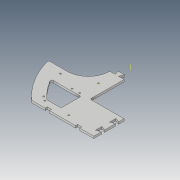
# Autodesk Inventor part: BR_topPlate
Saved by Autodesk Inventor 2018 (Build 220112000, 112)
## iProperties
Created: 2020-01-08
Part Number: BR_topPlate
Material: Generic
Document SubType Name: Modeling
Designer: anirudh
Density: 1 g/cm^3
Appearance: Default
Author: anirudh
Autodesk Inventor part; units mm, degrees
ref_plane "YZ Plane" through (0, 0, 0) normal (1, 0, 0) x (0, 1, 0)
ref_plane "XZ Plane" through (0, 0, 0) normal (0, 1, 0) x (-1, 0, 0)
ref_plane "XY Plane" through (0, 0, 0) normal (0, 0, 1) x (1, 0, 0)
sketch "Sketch1" plane through (0, 0, 0) normal (0, 1, 0) x (-1, 0, 0)
  line L0 (-159.8042, -152.4) -> (-128.1081, -152.4)
  line L1 (-159.8042, -152.4) -> (-128.1081, -152.4)
  line L2 (-128.1081, -147.32) -> (-117.9481, -147.32)
  line L3 (-128.1081, -152.4) -> (-128.1081, -147.32)
  line L4 (-117.9481, -147.32) -> (-117.9481, -152.4)
  line L5 (-128.1081, -147.32) -> (-117.9481, -147.32)
  line L6 (-117.9481, -152.4) -> (-55.88, -152.4)
  line L7 (-117.9481, -147.32) -> (-117.9481, -152.4)
  line L8 (-117.9481, -152.4) -> (-55.88, -152.4)
  line L9 (-55.88, -147.32) -> (-45.72, -147.32)
  line L10 (-55.88, -152.4) -> (-55.88, -147.32)
  line L11 (-45.72, -147.32) -> (-45.72, -152.4)
  line L12 (-55.88, -147.32) -> (-45.72, -147.32)
  line L13 (-45.72, -152.4) -> (20.32, -152.4)
  line L14 (-45.72, -147.32) -> (-45.72, -152.4)
  line L15 (-45.72, -152.4) -> (20.32, -152.4)
  line L16 (20.32, -147.32) -> (30.48, -147.32)
  line L17 (20.32, -152.4) -> (20.32, -147.32)
  line L18 (30.48, -147.32) -> (30.48, -152.4)
  line L19 (20.32, -147.32) -> (30.48, -147.32)
  line L20 (30.48, -147.32) -> (30.48, -152.4)
  line L21 (30.48, -152.4) -> (92.5481, -152.4)
  line L22 (30.48, -152.4) -> (92.5481, -152.4)
  line L23 (92.5481, -147.32) -> (102.7081, -147.32)
  line L24 (92.5481, -152.4) -> (92.5481, -147.32)
  line L25 (102.7081, -147.32) -> (102.7081, -152.4)
  line L26 (92.5481, -147.32) -> (102.7081, -147.32)
  line L27 (102.7081, -147.32) -> (102.7081, -152.4)
  arc A0 (134.4042, -152.4) -> (195.6623, -54.8317) centre (0, 0) ccw
  line L28 (102.7081, -152.4) -> (134.4042, -152.4)
  arc A1 (-221.0623, -54.8317) -> (-159.8042, -152.4) centre (-25.4, 0) ccw
  line L29 (134.4042, 152.4) -> (102.7081, 152.4)
  line L30 (134.4042, 152.4) -> (102.7081, 152.4)
  line L31 (-128.1081, 152.4) -> (-159.8042, 152.4)
  line L32 (-128.1081, 147.32) -> (-128.1081, 152.4)
  line L33 (-159.8042, 152.4) -> (-128.1081, 152.4)
  line L34 (-117.9481, 147.32) -> (-128.1081, 147.32)
  line L35 (-128.1081, 152.4) -> (-128.1081, 147.32)
  line L36 (-128.1081, 147.32) -> (-117.9481, 147.32)
  line L37 (-55.88, 152.4) -> (-117.9481, 152.4)
  line L38 (-117.9481, 147.32) -> (-117.9481, 152.4)
  line L39 (-55.88, 147.32) -> (-55.88, 152.4)
  line L40 (-117.9481, 152.4) -> (-55.88, 152.4)
  line L41 (-45.72, 147.32) -> (-55.88, 147.32)
  line L42 (-55.88, 152.4) -> (-55.88, 147.32)
  line L43 (-55.88, 147.32) -> (-45.72, 147.32)
  line L44 (20.32, 152.4) -> (-45.72, 152.4)
  line L45 (-45.72, 147.32) -> (-45.72, 152.4)
  line L46 (-45.72, 152.4) -> (20.32, 152.4)
  line L47 (30.48, 147.32) -> (20.32, 147.32)
  line L48 (20.32, 152.4) -> (20.32, 147.32)
  line L49 (20.32, 147.32) -> (30.48, 147.32)
  line L50 (30.48, 152.4) -> (30.48, 147.32)
  line L51 (30.48, 147.32) -> (30.48, 152.4)
  line L52 (92.5481, 147.32) -> (92.5481, 152.4)
  line L53 (30.48, 152.4) -> (92.5481, 152.4)
  line L54 (92.5481, 152.4) -> (92.5481, 147.32)
  line L55 (102.7081, 152.4) -> (102.7081, 147.32)
  line L56 (92.5481, 147.32) -> (102.7081, 147.32)
  line L57 (102.7081, 147.32) -> (102.7081, 152.4)
  arc A2 (-177.8, -50.8) -> (-177.8, 50.8) centre (-177.8, 0) ccw
  arc A3 (-177.8, -50.8) -> (-177.8, 50.8) centre (-177.8, 0) ccw
  arc A4 (152.4, 50.8) -> (152.4, -50.8) centre (152.4, 0) ccw
  arc A5 (152.4, 50.8) -> (152.4, -50.8) centre (152.4, 0) ccw
  line L58 (152.4, -50.8) -> (196.7476, -50.8)
  line L59 (152.4, 50.8) -> (196.7476, 50.8)
  line L60 (-177.8, -50.8) -> (-218.005, -50.8)
  line L61 (-177.8, -50.8) -> (-222.1476, -50.8)
  line L62 (-218.005, 50.8) -> (-177.8, 50.8)
  line L63 (-177.8, 50.8) -> (-222.1476, 50.8)
  arc A6 (-159.8042, 152.4) -> (-222.1476, 50.8) centre (-25.4, 0) ccw
  arc A7 (-222.1476, -50.8) -> (-159.8042, -152.4) centre (-25.4, 0) ccw
  arc A8 (134.4042, -152.4) -> (196.7476, -50.8) centre (0, 0) ccw
  arc A9 (196.7476, 50.8) -> (134.4042, 152.4) centre (0, 0) ccw
  line L64 (-12.7, -80.645) -> (-93.345, -80.645)
  line L65 (-93.345, -80.645) -> (67.945, -80.645)
  line L66 (67.945, -80.645) -> (67.945, 80.645)
  line L67 (67.945, 80.645) -> (-93.345, 80.645)
  line L68 (-93.345, 80.645) -> (-93.345, -80.645)
  circle A10 centre (-177.8, -63.5) radius 1.75
  circle A11 centre (-177.8, -63.5) radius 1.75
  circle A12 centre (-177.8, 63.5) radius 1.75
  circle A13 centre (-177.8, 63.5) radius 1.75
  circle A14 centre (-136.1822, -80.3402) radius 1.75
  circle A15 centre (-136.1822, -80.3402) radius 1.75
  circle A16 centre (-118.4022, -80.3402) radius 1.75
  circle A17 centre (-118.4022, -80.3402) radius 1.75
  circle A18 centre (-136.1822, 80.3402) radius 1.75
  circle A19 centre (-136.1822, 80.3402) radius 1.75
  circle A20 centre (-118.4022, 80.3402) radius 1.75
  circle A21 centre (-118.4022, 80.3402) radius 1.75
  circle A22 centre (93.0022, -80.3402) radius 1.75
  circle A23 centre (93.0022, -80.3402) radius 1.75
  circle A24 centre (110.7822, -80.3402) radius 1.75
  circle A25 centre (110.7822, -80.3402) radius 1.75
  circle A26 centre (152.4, -63.5) radius 1.75
  circle A27 centre (152.4, -63.5) radius 1.75
  circle A28 centre (152.4, 63.5) radius 1.75
  circle A29 centre (152.4, 63.5) radius 1.75
  circle A30 centre (93.0022, 80.3402) radius 1.75
  circle A31 centre (93.0022, 80.3402) radius 1.75
  circle A32 centre (110.7822, 80.3402) radius 1.75
  circle A33 centre (110.7822, 80.3402) radius 1.75
  dimension "d4" = 80.645
  dimension "d5" = 161.29
  constraints: 139 end point, 34 centre point, 30 perpendicular, 22 point on circle, 16 coincident, 6 horizontal, 4 collinear, 4 point on line, 2 parallel, 2 tangent
  measures "d4" distance of L64.start L64.end
  measures "d5" distance of L68.start L67.start
extrude "Extrusion1" add sketch "Sketch1" along normal blind 5.08
fillet "Fillet1" radius 3.175 8 edges at (222.1476, 2.54, 50.8) (222.1476, 2.54, -50.8) (93.345, 2.54, 80.645) (93.345, 2.54, -80.645) (-67.945, 2.54, -80.645) (-67.945, 2.54, 80.645) (-196.7476, 2.54, 50.8) (-196.7476, 2.54, -50.8)
sketch "Sketch2" plane through (0, 5.08, 0) normal (0, 1, 0) x (1, 0, 0)
  line L0 (-116.3974, -133.35) -> (-87.2998, -133.35)
  line L1 (-116.3974, -133.35) -> (-87.2998, -133.35)
  line L2 (-84.1248, -130.175) -> (-84.1248, -89.2048)
  line L3 (-84.1248, -130.175) -> (-84.1248, -89.2048)
  line L4 (-87.2998, -86.0298) -> (-150.1213, -86.0298)
  line L5 (-87.2998, -86.0298) -> (-150.1213, -86.0298)
  arc A0 (-152.8507, -90.8267) -> (-118.5137, -132.5418) centre (0, 0) ccw
  arc A1 (-152.8507, -90.8267) -> (-118.5137, -132.5418) centre (0, 0) ccw
  arc A2 (-118.5137, -132.5418) -> (-116.3974, -133.35) centre (-116.3974, -130.175) ccw
  arc A3 (-118.5137, -132.5418) -> (-116.3974, -133.35) centre (-116.3974, -130.175) ccw
  arc A4 (-87.2998, -133.35) -> (-84.1248, -130.175) centre (-87.2998, -130.175) ccw
  arc A5 (-87.2998, -133.35) -> (-84.1248, -130.175) centre (-87.2998, -130.175) ccw
  arc A6 (-84.1248, -89.2048) -> (-87.2998, -86.0298) centre (-87.2998, -89.2048) ccw
  arc A7 (-84.1248, -89.2048) -> (-87.2998, -86.0298) centre (-87.2998, -89.2048) ccw
  arc A8 (-150.1213, -86.0298) -> (-152.8507, -90.8267) centre (-150.1213, -89.2048) ccw
  arc A9 (-150.1213, -86.0298) -> (-152.8507, -90.8267) centre (-150.1213, -89.2048) ccw
  arc A10 (-152.4, -50.8) -> (-152.4, 50.8) centre (-152.4, 0) ccw
  arc A11 (177.8, 50.8) -> (177.8, -50.8) centre (177.8, 0) ccw
  line L6 (141.7974, -133.35) -> (112.6998, -133.35)
  line L7 (141.7974, -133.35) -> (112.6998, -133.35)
  line L8 (109.5248, -130.175) -> (109.5248, -89.2048)
  line L9 (109.5248, -130.175) -> (109.5248, -89.2048)
  line L10 (112.6998, -86.0298) -> (175.5213, -86.0298)
  line L11 (112.6998, -86.0298) -> (175.5213, -86.0298)
  arc A12 (112.6998, -86.0298) -> (109.5248, -89.2048) centre (112.6998, -89.2048) ccw
  arc A13 (112.6998, -86.0298) -> (109.5248, -89.2048) centre (112.6998, -89.2048) ccw
  arc A14 (178.2507, -90.8267) -> (175.5213, -86.0298) centre (175.5213, -89.2048) ccw
  arc A15 (178.2507, -90.8267) -> (175.5213, -86.0298) centre (175.5213, -89.2048) ccw
  arc A16 (109.5248, -130.175) -> (112.6998, -133.35) centre (112.6998, -130.175) ccw
  arc A17 (109.5248, -130.175) -> (112.6998, -133.35) centre (112.6998, -130.175) ccw
  arc A18 (143.9137, -132.5418) -> (178.2507, -90.8267) centre (25.4, 0) ccw
  arc A19 (143.9137, -132.5418) -> (178.2507, -90.8267) centre (25.4, 0) ccw
  arc A20 (141.7974, -133.35) -> (143.9137, -132.5418) centre (141.7974, -130.175) ccw
  arc A21 (141.7974, -133.35) -> (143.9137, -132.5418) centre (141.7974, -130.175) ccw
  arc A22 (-152.4, -50.8) -> (-152.4, 50.8) centre (-152.4, 0) ccw projected
  arc A23 (177.8, 50.8) -> (177.8, -50.8) centre (177.8, 0) ccw projected
  line L12 (-116.3974, 133.35) -> (-87.2998, 133.35)
  line L13 (-116.3974, 133.35) -> (-87.2998, 133.35)
  line L14 (-84.1248, 130.175) -> (-84.1248, 89.2048)
  line L15 (-84.1248, 130.175) -> (-84.1248, 89.2048)
  line L16 (-87.2998, 86.0298) -> (-150.1213, 86.0298)
  line L17 (-87.2998, 86.0298) -> (-150.1213, 86.0298)
  arc A24 (-118.5137, 132.5418) -> (-152.8507, 90.8267) centre (0, 0) ccw
  arc A25 (-118.5137, 132.5418) -> (-152.8507, 90.8267) centre (0, 0) ccw
  arc A26 (-116.3974, 133.35) -> (-118.5137, 132.5418) centre (-116.3974, 130.175) ccw
  arc A27 (-116.3974, 133.35) -> (-118.5137, 132.5418) centre (-116.3974, 130.175) ccw
  arc A28 (-84.1248, 130.175) -> (-87.2998, 133.35) centre (-87.2998, 130.175) ccw
  arc A29 (-84.1248, 130.175) -> (-87.2998, 133.35) centre (-87.2998, 130.175) ccw
  arc A30 (-87.2998, 86.0298) -> (-84.1248, 89.2048) centre (-87.2998, 89.2048) ccw
  arc A31 (-87.2998, 86.0298) -> (-84.1248, 89.2048) centre (-87.2998, 89.2048) ccw
  arc A32 (-152.8507, 90.8267) -> (-150.1213, 86.0298) centre (-150.1213, 89.2048) ccw
  arc A33 (-152.8507, 90.8267) -> (-150.1213, 86.0298) centre (-150.1213, 89.2048) ccw
  line L18 (141.7974, 133.35) -> (112.6998, 133.35)
  line L19 (141.7974, 133.35) -> (112.6998, 133.35)
  line L20 (109.5248, 130.175) -> (109.5248, 89.2048)
  line L21 (109.5248, 130.175) -> (109.5248, 89.2048)
  line L22 (112.6998, 86.0298) -> (175.5213, 86.0298)
  line L23 (112.6998, 86.0298) -> (175.5213, 86.0298)
  arc A34 (109.5248, 89.2048) -> (112.6998, 86.0298) centre (112.6998, 89.2048) ccw
  arc A35 (109.5248, 89.2048) -> (112.6998, 86.0298) centre (112.6998, 89.2048) ccw
  arc A36 (175.5213, 86.0298) -> (178.2507, 90.8267) centre (175.5213, 89.2048) ccw
  arc A37 (175.5213, 86.0298) -> (178.2507, 90.8267) centre (175.5213, 89.2048) ccw
  arc A38 (112.6998, 133.35) -> (109.5248, 130.175) centre (112.6998, 130.175) ccw
  arc A39 (112.6998, 133.35) -> (109.5248, 130.175) centre (112.6998, 130.175) ccw
  arc A40 (178.2507, 90.8267) -> (143.9137, 132.5418) centre (25.4, 0) ccw
  arc A41 (178.2507, 90.8267) -> (143.9137, 132.5418) centre (25.4, 0) ccw
  arc A42 (143.9137, 132.5418) -> (141.7974, 133.35) centre (141.7974, 130.175) ccw
  arc A43 (143.9137, 132.5418) -> (141.7974, 133.35) centre (141.7974, 130.175) ccw
  point P0 (0, 0)
  point P1 (25.4, 0)
  constraints: 84 point on circle, 48 end point, 42 centre point, 20 coincident, 2 collinear, 1 horizontal
extrude "Extrusion2" cut sketch "Sketch2" against normal blind 5.08
sketch "Sketch4" plane through (0, 5.08, 0) normal (0, 1, 0) x (1, 0, 0)
  circle A0 centre (-152.4, -63.5) radius 1.75 projected
  line L0 (-152.4, -50.8) -> (-192.605, -50.8) projected
  arc A1 (-195.6623, -54.8317) -> (-134.4042, -152.4) centre (0, 0) ccw projected
  circle A2 centre (-184.3483, -57.15) radius 1.75
  circle A3 centre (-163.0494, -57.15) radius 1.75
  circle A4 centre (-152.4, 63.5) radius 1.75 projected
  line L1 (-192.605, 50.8) -> (-152.4, 50.8) projected
  arc A5 (-134.4042, 152.4) -> (-195.6623, 54.8317) centre (0, 0) ccw projected
  circle A6 centre (-184.3483, 57.15) radius 1.75
  circle A7 centre (-163.0494, 57.15) radius 1.75
  line L2 (-64.77, 80.645) -> (90.17, 80.645) projected
  line L3 (12.7, 80.645) -> (12.7, 167.4732)
  line L4 (12.7, 167.4732) -> (12.7, -184.4325)
  circle A8 centre (100.7872, -56.769) radius 1.75
  circle A9 centre (100.7872, 56.769) radius 1.75
  circle A10 centre (187.4774, -56.769) radius 1.75
  circle A11 centre (187.4774, 56.769) radius 1.75
  dimension "d11" = 3.5
  dimension "d12" = 3.5
  dimension "d13" = 3.5
  dimension "d14" = 3.5
  dimension "d67" = 3.5
  dimension "d70" = 3.5
  dimension "d73" = 3.5
  dimension "d74" = 3.5
  constraints: 8 centre point, 4 end point, 1 midpoint, 1 point on line, 1 vertical
  measures "d11" diameter of A2
  measures "d12" diameter of A3
  measures "d13" diameter of A6
  measures "d14" diameter of A7
  measures "d67" diameter of A8
  measures "d70" diameter of A9
  measures "d73" diameter of A10
  measures "d74" diameter of A11
sketch "Sketch5" plane through (0, 5.08, 0) normal (0, 1, 0) x (1, 0, 0)
  line L0 (109.5248, 89.2048) -> (109.5248, 130.175) projected
  line L1 (-84.1248, 130.175) -> (-84.1248, 89.2048) projected
  line L2 (-92.5481, -152.4) -> (-30.48, -152.4) projected
  line L3 (-84.1248, -89.2048) -> (-84.1248, -130.175) projected
  circle A0 centre (85.3186, -139.312) radius 1.75
  circle A1 centre (12.7, -141.0532) radius 1.75
  circle A2 centre (-59.9186, -139.312) radius 1.75
  circle A3 centre (85.3186, 139.312) radius 1.75
  circle A4 centre (12.7, 139.312) radius 1.75
  circle A5 centre (-59.9186, 139.312) radius 1.75
  point P0 (0, 0)
  point P1 (55.88, 147.32)
  dimension "d55" = 3.5
  dimension "d56" = 3.5
  dimension "d57" = 3.5
  dimension "d62" = 3.5
  dimension "d64" = 3.5
  constraints: 6 centre point
  measures "d55" diameter of A0
  measures "d56" diameter of A1
  measures "d57" diameter of A2
  measures "d62" diameter of A3
  measures "d64" diameter of A5
extrude "Extrusion5" cut sketch "Sketch5" against normal blind 25.4
sketch "Sketch7" plane through (0, 5.08, 0) normal (0, 1, 0) x (1, 0, 0)
  line L0 (93.345, 77.47) -> (93.345, -77.47) projected
  line L1 (-67.945, 77.47) -> (-67.945, -77.47) projected
  circle A0 centre (-90.445, -38.1) radius 1.75
  circle A1 centre (-90.445, 0) radius 1.75
  circle A2 centre (-90.445, 38.1) radius 1.75
  point P0 (0, 0)
  dimension "d44" = 3.5
  constraints: 3 centre point
  measures "d44" diameter of A0
extrude "Extrusion6" cut sketch "Sketch7" against normal blind 25.4
ref_plane "Work Plane4" through (-59.9186, 5.08, 139.312) normal (-0.0239699, 0, 0.9997127) x (0, -1, 0)
ref_plane "Work Plane5" through (-59.9186, 5.08, -139.312) normal (0, 0, 1) x (0, -1, 0)
ref_plane "Work Plane6" through (12.7, 5.08, -139.312) normal (-1, 0, 0) x (0, -1, 0)
ref_plane "Work Plane7" through (-90.445, 5.08, 38.1) normal (1, 0, 0) x (0, -1, 0)
ref_plane "Work Plane8" through (-152.4, 0, 0) normal (0, 0, -1) x (0, 1, 0)
sketch "Sketch11" plane through (0, 5.08, 0) normal (0, 1, 0) x (1, 0, 0)
  circle A0 centre (180.7464, 63.5) radius 1.75
  circle A1 centre (180.7464, -63.5) radius 1.75
  circle A2 centre (-155.3464, 63.5) radius 1.75
  circle A3 centre (-155.3464, -63.5) radius 1.75
  point P0 (0, 0)
  point P1 (177.8, 63.5)
  dimension "d78" = 3.5
  dimension "d80" = 3.5
  dimension "d82" = 3.5
  dimension "d84" = 3.5
  constraints: 4 centre point
  measures "d78" diameter of A0
  measures "d80" diameter of A1
  measures "d82" diameter of A2
  measures "d84" diameter of A3
sketch "Sketch12" plane through (0, 5.08, 0) normal (0, 1, 0) x (1, 0, 0)
  circle A0 centre (177.8, 63.5) radius 4.4542
  circle A1 centre (177.8, -63.5) radius 3.6803
  circle A2 centre (-152.4, 63.5) radius 4.3114
  circle A3 centre (-152.4, -63.5) radius 4.653
  point P0 (0, 0)
  constraints: 4 centre point, 4 coincident
extrude "Extrusion8" add sketch "Sketch12" against normal blind 5.08
extrude "Extrusion9" cut sketch "Sketch11" against normal blind 25.4
sketch "Sketch13" plane through (0, 5.08, 0) normal (0, 1, 0) x (1, 0, 0)
  line L0 (93.345, -51.689) -> (194.945, -51.689)
  line L1 (194.945, -51.689) -> (194.945, 51.689)
  line L2 (194.945, 51.689) -> (93.345, 51.689)
  line L3 (93.345, 51.689) -> (93.345, -51.689)
  circle A0 centre (100.7999, -46.609) radius 1.75
  circle A1 centre (100.7999, 46.609) radius 1.75
  circle A2 centre (187.4901, -46.609) radius 1.75
  circle A3 centre (187.4901, 46.609) radius 1.75
  line L4 (93.345, 0) -> (73.1184, 0)
  line L5 (93.345, 0) -> (83.2317, 0)
  line L6 (194.945, -51.689) -> (194.945, -41.529)
  line L7 (194.945, -41.529) -> (144.145, -41.529)
  line L8 (144.145, -41.529) -> (144.145, -51.689)
  line L9 (194.945, 51.689) -> (194.945, 41.529)
  line L10 (194.945, 41.529) -> (144.145, 41.529)
  line L11 (144.145, 41.529) -> (144.145, 51.689)
  point P0 (0, 0)
  point P1 (93.345, -77.47)
  point P2 (93.345, 77.47)
  constraints: 24 end point, 4 centre point, 4 midpoint, 3 perpendicular, 2 horizontal, 2 parallel, 2 point on line
sketch "Sketch14" plane through (0, 5.08, 0) normal (0, 1, 0) x (1, 0, 0)
  line L0 (93.345, 0) -> (73.1184, 0)
  line L1 (93.345, 0) -> (83.2317, 0)
  line L2 (194.945, -51.689) -> (194.945, -41.529)
  line L3 (194.945, -41.529) -> (144.145, -41.529)
  line L4 (144.145, -41.529) -> (144.145, -51.689)
  line L5 (194.945, 51.689) -> (194.945, 41.529)
  line L6 (194.945, 41.529) -> (144.145, 41.529)
  line L7 (144.145, 41.529) -> (144.145, 51.689)
  line L8 (144.145, -51.689) -> (194.945, -51.689)
  line L9 (144.145, 51.689) -> (194.945, 51.689)
  point P0 (0, 0)
  constraints: 20 end point, 2 horizontal, 1 midpoint, 1 parallel, 1 perpendicular
extrude "Extrusion10" add sketch "Sketch14" against normal blind 5.08
fillet "Fillet2" radius 3.175 6 edges at (194.945, 2.54, 50.8) (194.945, 2.54, 41.529) (148.5428, 2.54, 41.529) (148.5428, 2.54, -41.529) (194.945, 2.54, -41.529) (194.945, 2.54, -50.8)
extrude "Extrusion11" cut sketch "Sketch13" against normal blind 6.35 contours A0 | A1 | A2 | A3
sketch "Sketch15" plane through (0, 5.08, 0) normal (0, 1, 0) x (1, 0, 0)
  circle A0 centre (153.6294, 130.175) radius 1.75
  circle A1 centre (143.9546, 137.541) radius 1.75
  arc A2 (147.6846, 40.9109) -> (147.6846, -40.9109) centre (177.8, 0) ccw projected
  arc A3 (-152.4, -50.8) -> (-152.4, 50.8) centre (-152.4, 0) ccw projected
  line L0 (177.8, 0) -> (-152.4, 0)
  line L1 (12.7, 0) -> (12.7, -206.6585)
  circle A4 centre (153.6294, -130.175) radius 1.75
  circle A5 centre (143.9546, -137.541) radius 1.75
  circle A6 centre (-128.2294, 130.175) radius 1.75
  circle A7 centre (-118.5546, 137.541) radius 1.75
  circle A8 centre (-128.2294, -130.175) radius 1.75
  circle A9 centre (-118.5546, -137.541) radius 1.75
  point P0 (0, 0)
  point P1 (128.1081, 152.4)
  point P2 (143.9137, 132.5418)
  point P3 (141.7974, 130.175)
  point P4 (143.9137, -132.5418)
  point P5 (141.7974, -130.175)
  point P6 (-118.5137, -132.5418)
  constraints: 9 symmetric about line, 8 centre point, 4 end point, 1 horizontal, 1 midpoint, 1 perpendicular, 6 other
extrude "Extrusion12" cut sketch "Sketch15" against normal blind 25.4
sketch "Sketch16" plane through (0, 5.08, 0) normal (0, 1, 0) x (1, 0, 0)
  circle A0 centre (12.7, 139.312) radius 1.75 projected
  circle A1 centre (12.7, 139.312) radius 1.75
  circle A2 centre (12.7, -141.0532) radius 1.75 projected
  circle A3 centre (12.7, -141.0532) radius 1.75
  point P0 (0, 0)
  constraints: 2 centre point, 2 coincident
extrude "Extrusion13" add sketch "Sketch16" against normal blind 5.08
sketch "Sketch17" plane through (0, 5.08, 0) normal (0, 1, 0) x (1, 0, 0)
  circle A0 centre (-90.445, 0) radius 1.75 projected
  circle A1 centre (-90.445, 0) radius 1.75
  point P0 (0, 0)
  constraints: 1 centre point, 1 coincident
extrude "Extrusion14" add sketch "Sketch17" against normal blind 5.08
sketch "Sketch18" plane through (0, 5.08, 0) normal (0, 1, 0) x (1, 0, 0)
  line L0 (128.1081, -152.4) -> (159.8042, -152.4) projected
  arc A0 (-195.6623, -54.8317) -> (-134.4042, -152.4) centre (0, 0) ccw projected
  line L1 (-20.32, -152.4) -> (45.72, -152.4) projected
  line L2 (45.72, 152.4) -> (-20.32, 152.4) projected
  line L3 (12.7, 0) -> (-238.1245, 0)
  line L4 (12.7, -152.4) -> (237.6065, -152.4)
  line L5 (237.6065, -152.4) -> (237.6065, 180.2856)
  line L6 (237.6065, 180.2856) -> (12.7, 180.2856)
  line L7 (-238.1245, 0) -> (12.7, 0)
  line L8 (12.7, 180.2856) -> (-238.1245, 180.2856)
  line L9 (-238.1245, 180.2856) -> (-238.1245, 0)
  line L10 (12.7, 0) -> (12.7, -152.4)
  constraints: 16 end point, 3 horizontal, 2 parallel, 1 midpoint, 1 perpendicular, 1 vertical
extrude "Extrusion15" cut sketch "Sketch18" against normal blind 5.08
sketch "Sketch19" plane through (0, 5.08, 0) normal (0, 1, 0) x (1, 0, 0)
  line L0 (2.54, -97.3138) -> (2.54, -104.9338)
  line L1 (2.54, -97.3138) -> (2.54, -89.6937)
  line L2 (12.7, -147.32) -> (12.7, -80.645)
  line L3 (12.7, -152.4) -> (12.7, -80.645)
  line L4 (12.7, -126.8413) -> (2.54, -123.0313)
  line L5 (12.7, -130.6513) -> (12.7, -126.8413)
  line L6 (2.54, -130.6513) -> (2.54, -123.0313)
  line L7 (12.7, -130.6513) -> (12.7, -134.4613)
  line L8 (2.54, -130.6513) -> (2.54, -138.2713)
  line L9 (12.7, -134.4613) -> (2.54, -138.2713)
  line L10 (12.7, -113.9825) -> (12.7, -147.32)
  line L11 (12.7, -97.3138) -> (12.7, -101.1238)
  line L12 (12.7, -97.3138) -> (12.7, -93.5038)
  line L13 (12.7, -93.5038) -> (2.54, -89.6937)
  line L14 (12.7, -113.9825) -> (12.7, -80.645)
  line L15 (12.7, -101.1238) -> (2.54, -104.9338)
  line L16 (12.7, -80.645) -> (12.7, -152.4)
  line L17 (-84.7725, 10.16) -> (-92.3925, 10.16)
  line L18 (-84.7725, 10.16) -> (-77.1525, 10.16)
  line L19 (-84.7725, 0) -> (-88.5825, 0)
  line L20 (-88.5825, 0) -> (-92.3925, 10.16)
  line L21 (-84.7725, 0) -> (-80.9625, 0)
  line L22 (-80.9625, 0) -> (-77.1525, 10.16)
  line L23 (-101.6, 0) -> (-67.945, 0) projected
  line L24 (-67.945, 0) -> (-101.6, 0)
  line L25 (2.54, -97.3138) -> (2.54, -104.9338)
  line L26 (2.54, -97.3138) -> (2.54, -89.6937)
  line L27 (12.7, -147.32) -> (12.7, -80.645)
  line L28 (12.7, -152.4) -> (12.7, -80.645)
  line L29 (12.7, -126.8413) -> (2.54, -123.0313)
  line L30 (12.7, -130.6513) -> (12.7, -126.8413)
  line L31 (2.54, -130.6513) -> (2.54, -123.0313)
  line L32 (12.7, -130.6513) -> (12.7, -134.4613)
  line L33 (2.54, -130.6513) -> (2.54, -138.2713)
  line L34 (12.7, -134.4613) -> (2.54, -138.2713)
  line L35 (12.7, -113.9825) -> (12.7, -147.32)
  line L36 (12.7, -97.3138) -> (12.7, -101.1238)
  line L37 (12.7, -97.3138) -> (12.7, -93.5038)
  line L38 (12.7, -93.5038) -> (2.54, -89.6937)
  line L39 (12.7, -113.9825) -> (12.7, -80.645)
  line L40 (12.7, -101.1238) -> (2.54, -104.9338)
  line L41 (12.7, -80.645) -> (12.7, -152.4)
  line L42 (-84.7725, 10.16) -> (-77.1525, 10.16)
  line L43 (-80.9625, 0) -> (-77.1525, 10.16)
  line L44 (-84.7725, 10.16) -> (-92.3925, 10.16)
  line L45 (-84.7725, 0) -> (-80.9625, 0)
  line L46 (-84.7725, 0) -> (-88.5825, 0)
  line L47 (-88.5825, 0) -> (-92.3925, 10.16)
  line L48 (-101.6, 0) -> (-67.945, 0)
  line L49 (-67.945, 0) -> (-101.6, 0)
  point P0 (0, 0)
  point P1 (0, 0)
  constraints: 98 end point, 6 collinear, 2 midpoint, 2 vertical
sketch "Sketch20" plane through (0, 5.08, 0) normal (0, 1, 0) x (1, 0, 0)
  line L0 (2.54, -97.3138) -> (2.54, -104.9338)
  line L1 (2.54, -97.3138) -> (2.54, -89.6937)
  line L2 (12.7, -147.32) -> (12.7, -80.645)
  line L3 (12.7, -152.4) -> (12.7, -80.645)
  line L4 (12.7, -126.8413) -> (2.54, -123.0313)
  line L5 (12.7, -130.6513) -> (12.7, -126.8413)
  line L6 (2.54, -130.6513) -> (2.54, -123.0313)
  line L7 (12.7, -130.6513) -> (12.7, -134.4613)
  line L8 (2.54, -130.6513) -> (2.54, -138.2713)
  line L9 (12.7, -134.4613) -> (2.54, -138.2713)
  line L10 (12.7, -113.9825) -> (12.7, -147.32)
  line L11 (12.7, -97.3138) -> (12.7, -101.1238)
  line L12 (12.7, -97.3138) -> (12.7, -93.5038)
  line L13 (12.7, -93.5038) -> (2.54, -89.6937)
  line L14 (12.7, -113.9825) -> (12.7, -80.645)
  line L15 (12.7, -101.1238) -> (2.54, -104.9338)
  line L16 (12.7, -80.645) -> (12.7, -152.4)
  line L17 (-84.7725, 10.16) -> (-77.1525, 10.16)
  line L18 (-80.9625, 0) -> (-77.1525, 10.16)
  line L19 (-84.7725, 10.16) -> (-92.3925, 10.16)
  line L20 (-84.7725, 0) -> (-80.9625, 0)
  line L21 (-84.7725, 0) -> (-88.5825, 0)
  line L22 (-88.5825, 0) -> (-92.3925, 10.16)
  line L23 (-101.6, 0) -> (-67.945, 0)
  line L24 (-67.945, 0) -> (-101.6, 0)
  line L25 (2.54, -97.3138) -> (2.54, -104.9338)
  line L26 (2.54, -97.3138) -> (2.54, -89.6937)
  line L27 (12.7, -147.32) -> (12.7, -80.645)
  line L28 (12.7, -152.4) -> (12.7, -80.645)
  line L29 (12.7, -126.8413) -> (2.54, -123.0313)
  line L30 (12.7, -130.6513) -> (12.7, -126.8413)
  line L31 (2.54, -130.6513) -> (2.54, -123.0313)
  line L32 (12.7, -130.6513) -> (12.7, -134.4613)
  line L33 (2.54, -130.6513) -> (2.54, -138.2713)
  line L34 (12.7, -134.4613) -> (2.54, -138.2713)
  line L35 (12.7, -113.9825) -> (12.7, -147.32)
  line L36 (12.7, -97.3138) -> (12.7, -101.1238)
  line L37 (12.7, -97.3138) -> (12.7, -93.5038)
  line L38 (12.7, -93.5038) -> (2.54, -89.6937)
  line L39 (12.7, -113.9825) -> (12.7, -80.645)
  line L40 (12.7, -101.1238) -> (2.54, -104.9338)
  line L41 (12.7, -80.645) -> (12.7, -152.4)
  line L42 (-84.7725, 10.16) -> (-77.1525, 10.16)
  line L43 (-80.9625, 0) -> (-77.1525, 10.16)
  line L44 (-84.7725, 10.16) -> (-92.3925, 10.16)
  line L45 (-84.7725, 0) -> (-80.9625, 0)
  line L46 (-84.7725, 0) -> (-88.5825, 0)
  line L47 (-88.5825, 0) -> (-92.3925, 10.16)
  line L48 (-101.6, 0) -> (-67.945, 0)
  line L49 (-67.945, 0) -> (-101.6, 0)
  point P0 (0, 0)
  point P1 (0, 0)
  point P2 (0, 0)
  constraints: 100 end point, 6 collinear, 2 midpoint, 2 vertical
extrude "Extrusion16" add sketch "Sketch19" against normal blind 5.08 contours L18 L22 L21 L19 L20 L17
extrude "Extrusion17" cut sketch "Sketch20" against normal blind 5.08 contours L1 L13 L2 L15 L0 | L9 L8 L6 L4 L2
body "Solid1"
